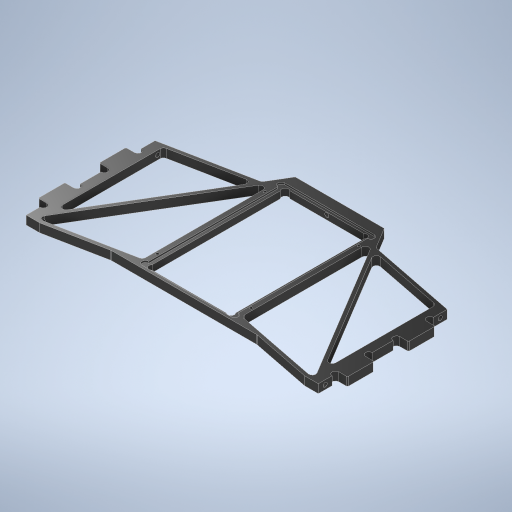
# Autodesk Inventor part: TorsoLowerFrame
Saved by Autodesk Inventor 2024.2 (Build 282272000, 272)
## iProperties
Created: 2024-01-11
Part Number: TorsoLowerFrame
Material: Aluminum 2014-T4
Document SubType Name: Modeling
Designer: Masato Kubotera
Density: 2.8 g/cm^3
Appearance: Glossy - Black
Vendor: meviy
Mass: 47.2837 g
Surface Area: 169.328 cm^2
Volume: 16.887 cm^3
Author: Masato Kubotera
Autodesk Inventor part; units mm, degrees
ref_plane "YZ Plane" through (0, 0, 0) normal (1, 0, 0) x (0, 1, 0)
ref_plane "XZ Plane" through (0, 0, 0) normal (0, 1, 0) x (-1, 0, 0)
sketch "Sketch1" plane through (0, 0, 0) normal (0, 0, 1) x (1, 0, 0)
  line L0 (-53, -85) -> (37.5, -85) construction
  line L1 (37.5, 85) -> (-53, 85) construction
  line L2 (0, -85) -> (0, 85) construction
  line L3 (-53, 0) -> (37.5, 0)
  line L4 (10, 90) -> (25.5, 90)
  line L5 (10, 90) -> (10, 85)
  arc A0 (6, 85) -> (10, 85) centre (8, 85) ccw
  line L6 (37.5, 85) -> (37.5, -85) construction
  line L7 (-53, -85) -> (-53, 85) construction
  line L8 (28.85, -25.8) -> (-53.75, -25.8) construction
  line L9 (-53.75, -25.8) -> (-53.75, 25.8) construction
  line L10 (-53.75, 25.8) -> (28.85, 25.8) construction
  line L11 (28.85, 25.8) -> (28.85, -25.8) construction
  line L12 (28.85, -25.8) -> (-53.75, 25.8) construction
  line L13 (-53.75, -25.8) -> (28.85, 25.8) construction
  line L14 (29.1, -26.05) -> (-54, -26.05)
  line L15 (-54, -26.05) -> (-54, 26.05)
  line L16 (-54, 26.05) -> (29.1, 26.05)
  line L17 (29.1, 26.05) -> (29.1, -26.05)
  line L18 (29.1, -26.05) -> (-54, 26.05) construction
  line L19 (-54, -26.05) -> (29.1, 26.05) construction
  line L20 (-52.5, 24.3) -> (27.6, 24.3) construction
  line L21 (27.6, 24.3) -> (27.6, -24.3) construction
  line L22 (27.6, -24.3) -> (-52.5, -24.3)
  line L23 (-52.5, -24.3) -> (-52.5, 24.3) construction
  line L24 (-52.5, 24.3) -> (27.6, -24.3) construction
  line L25 (27.6, 24.3) -> (-52.5, -24.3) construction
  line L26 (26.1724, 30.4098) -> (35.4616, 77.1098)
  line L27 (32.4688, 79.2137) -> (-45.1376, 32.5137)
  line L28 (-44.1064, 28.8) -> (24.2108, 28.8)
  line L29 (21.8631, 79.5) -> (-34.9135, 79.5)
  line L30 (37.5, 27.3) -> (-50.7865, 27.3) construction
  arc A1 (24.2108, 28.8) -> (26.1724, 30.4098) centre (24.2108, 30.8) ccw
  arc A2 (-45.1376, 32.5137) -> (-44.1064, 28.8) centre (-44.1064, 30.8) ccw
  arc A3 (22.8943, 75.7863) -> (21.8631, 79.5) centre (21.8631, 77.5) ccw
  arc A4 (29.1, 26.05) -> (25.1, 26.05) centre (27.1, 26.05) ccw
  arc A5 (27.6, 21.4716) -> (24.7716, 24.3) centre (26.1858, 22.8858) ccw
  arc A6 (-49.6716, 24.3) -> (-52.5, 21.4716) centre (-51.0858, 22.8858) ccw
  arc A7 (-50, 26.05) -> (-54, 26.05) centre (-52, 26.05) ccw
  circle A8 centre (18.85, 27.3) radius 1.5 construction
  circle A9 centre (18.85, 27.3) radius 1 construction
  line L31 (-12.45, -25.8) -> (-12.45, 25.7819) construction
  circle A10 centre (-43.75, 27.3) radius 1.5 construction
  circle A11 centre (-43.75, 27.3) radius 1 construction
  circle A12 centre (18.85, 27.3) radius 2.5 construction
  circle A13 centre (-43.75, 27.3) radius 2.5 construction
  line L32 (17.75, 90) -> (17.75, 85) construction
  line L33 (25.5, 90) -> (25.5, 85)
  arc A14 (25.5, 85) -> (29.5, 85) centre (27.5, 85) ccw
  line L34 (37.5, 85) -> (29.5, 85)
  line L35 (-10, 90) -> (-25.5, 90)
  line L36 (-10, 90) -> (-10, 85)
  arc A15 (-10, 85) -> (-6, 85) centre (-8, 85) ccw
  line L37 (-17.75, 90) -> (-17.75, 85) construction
  line L38 (-25.5, 90) -> (-25.5, 85)
  arc A16 (-29.5, 85) -> (-25.5, 85) centre (-27.5, 85) ccw
  line L39 (6, 85) -> (-6, 85)
  line L40 (33.5, 85) -> (33.5, 79) construction
  line L41 (-33.5, 85) -> (-33.5, 79) construction
  line L42 (-44.5951, 39.0791) -> (-36.875, 77.8902)
  line L43 (-41.6023, 36.9752) -> (22.8943, 75.7863)
  line L44 (-37.5, 85) -> (-29.5, 85)
  arc A17 (-44.5951, 39.0791) -> (-41.6023, 36.9752) centre (-42.6335, 38.6889) ccw
  arc A18 (-34.9135, 79.5) -> (-36.875, 77.8902) centre (-34.9135, 77.5) ccw
  line L45 (27.6, 0) -> (27.6, 21.4716)
  line L46 (24.7716, 24.3) -> (-49.6716, 24.3)
  line L47 (-52.5, 21.4716) -> (-52.5, 0)
  line L48 (-37.5, 85) -> (-47.6213, 34.1169)
  arc A19 (35.4616, 77.1098) -> (32.4688, 79.2137) centre (33.5, 77.5) ccw
  line L49 (-60, 25.9043) -> (-60, 0)
  line L50 (-60, 0) -> (-53, 0)
  line L51 (-60, 39.2) -> (-48.5, 39.2) construction
  line L52 (-48.5, 39.2) -> (-48.5, 44.2) construction
  line L53 (-48.5, 44.2) -> (-60, 44.2) construction
  line L54 (29.1, 26.05) -> (29.1, 20.1473)
  line L55 (-60, 25.9043) -> (-48.5516, 32.7934)
  line L56 (30.6, 0) -> (30.6, 42.2204)
  arc A20 (30.6384, 42.6106) -> (30.6, 42.2204) centre (32.6, 42.2204) ccw
  line L57 (37.5, 85) -> (37.5, 77.106)
  line L58 (37.5, 77.106) -> (30.6384, 42.6106)
  arc A21 (-48.5516, 32.7934) -> (-47.6213, 34.1169) centre (-49.5828, 34.5071) ccw
  point P0 (0, 0)
  point P1 (50, -85)
  point P2 (-47, 0)
  point P3 (-12.45, 0)
  point P4 (-49.0507, 0)
  point P5 (29.1, 0)
  point P6 (-20.5577, 28.8)
  point P7 (-52.5, 0)
  point P8 (27.6, 0)
  point P9 (24.6, 26.05)
  point P10 (-45.4774, 34.6434)
  point P11 (-36.5548, 79.5)
  point P12 (-52.5, 0)
  point P13 (27.6, 0)
  point P14 (0, 85)
  point P15 (-48.8888, 27.7448)
  point P16 (-60, 26.05)
  point P17 (-60, 24.5149)
  point P18 (-47.7938, 33.2495)
  point P19 (-54, 0)
  point P20 (-57, 0)
  dimension "d1" = 170
  dimension "d2" = 2
  dimension "d3" = 5
  dimension "d55" = 82.6
  dimension "d56" = 51.6
  dimension "d57" = 0.25
  dimension "d58" = 0.25
  dimension "d62" = 2
  dimension "d81" = 3
  dimension "d82" = 2
  dimension "d85" = 1.5
  dimension "d86" = 1.5
  dimension "d94" = 10
  dimension "d95" = 5
  dimension "d99" = 6
  dimension "d100" = 8
  dimension "d102" = 15.5
  dimension "d103" = 20
  dimension "d104" = 37.5
  dimension "d118" = 5.5
  dimension "d121" = 2
  dimension "d122" = 53
  dimension "d123" = 2
  dimension "d127" = 8.65
  dimension "d128" = 60
  dimension "d129" = 6
  dimension "d130" = 11.5
  dimension "d131" = 5
  dimension "d132" = 40.8
  dimension "d134" = 101.25
  dimension "d139" = 1.5
  dimension "d141" = 2
  dimension "d143" = 2
  constraints: 121 end point, 35 point on circle, 34 point on line, 22 centre point, 22 tangent, 20 symmetric about line, 15 midpoint, 11 equal radius, 10 horizontal, 10 parallel, 8 vertical, 5 coincident, 4 collinear, 3 perpendicular, 7 other
  measures "d1" distance of L1.start L0.end
  measures "d2" radius of A0
  measures "d3" distance of L4.start L5.end
  measures "d55" distance of L9.end L10.end
  measures "d56" distance of L8.end L9.end
  measures "d57" distance between parallel lines of L16 L10
  measures "d58" distance between parallel lines of L15 L9
  measures "d62" radius of A1
  measures "d81" diameter of A8
  measures "d82" diameter of A9
  measures "d85" distance between parallel lines of L10 L20
  measures "d86" distance between parallel lines of L21 L17
  measures "d94" horizontal distance of L10.end A8.centre
  measures "d95" diameter of A12
  measures "d99" distance of L40.start L40.end
  measures "d100" distance between parallel lines of L33 L40
  measures "d102" distance of L4.start L4.end
  measures "d103" distance between parallel lines of L36 L5
  measures "d104" distance between parallel lines of L6 L2
  measures "d118" distance between parallel lines of L1 L29
  measures "d121" distance between parallel lines of L42 L48
  measures "d122" distance of point (0, 85) L1.end
  measures "d123" distance between parallel lines of L27 L43
  measures "d127" distance between parallel lines of L6 L11
  measures "d128" distance between parallel lines of L49 L2
  measures "d129" distance between parallel lines of L15 L49
  measures "d130" distance of L51.start L51.end
  measures "d131" distance of L51.end L52.end
  measures "d132" distance between parallel lines of L53 L1
  measures "d134" angle of L42 L29
  measures "d139" distance between parallel lines of L56 L17
  measures "d141" distance between parallel lines of L58 L26
  measures "d143" distance edge to line of A19 L6
extrude "Extrusion1" add sketch "Sketch1" against normal blind 5 contours L50 L15 L16 L17 L3 L45 A5 L46 A6 L47 | L50 L49 L55 A21 L48 L44 A16 L38 L35 L36 A15 L39 A0 L5 L4 L33 A14 L34 L57 L58 A20 L56 L3 L17 A4 L16 A7 L15 | A7 L16 | A4 L16
extrude "Extrusion2" cut sketch "Sketch1" against normal blind 1 contours L50 L15 L16 L17 L3 L45 A5 L46 A6 L47 | L3 L17 L14 L15 L50 | L47 A6 L46 A5 L45 L3 | A7 L16 | A4 L16
hole "M2" at (18.85, 27.3, 0) at (-43.75, 27.3, 0) direction (0, 0, -1) diameter 1.567 end through all thread size "M2x0.4" class "6H" standard "ANSI Metric M Profile"
sketch "Sketch6" plane through (29.5, 85, 0) normal (0, 1, 0) x (1, 0, 0)
  line L0 (0, 5) -> (8, 5) projected
  line L1 (4, 5) -> (4, 0)
  line L2 (8, 0) -> (0, 0) projected
  line L3 (-63, 5) -> (-63, 0)
  line L4 (-67, 5) -> (-59, 5) projected
  point P0 (-29.5, 0)
  point P1 (-86, 5)
  point P2 (-86, 0)
  point P3 (4, 0)
  point P4 (-63, 0)
  point P5 (4, 2.5)
  point P6 (-63, 2.5)
  constraints: 4 end point, 4 midpoint, 2 vertical
hole "SideーM3" at (33.5, 85, -2.5) at (-33.5, 85, -2.5) direction (0, -1, 0) diameter 2.459 depth 10 thread size "M3x0.5" class "6H" standard "ANSI Metric M Profile"
chamfer "C0.5" distance 0.5 angle 45 4 edges at (25.5, 90, -2.5) (10, 90, -2.5) (-10, 90, -2.5) (-25.5, 90, -2.5)
mirror "Mirror5" about plane through (0, 0, 0) normal (0, 1, 0)
ref_plane "Work Plane1" through (-12.45, 21.4716, -1) normal (1, 0, 0) x (0, 0, -1)
sketch "Sketch7" plane through (-60, 25.9043, -5) normal (-1, 0, 0) x (0, 0, 1)
  line L0 (5, -25.9043) -> (0, -25.9043)
  line L1 (0, 0) -> (0, -51.8087) projected
  point P0 (2.5, -25.9043)
  point P1 (2.5, -25.9043)
  constraints: 2 end point, 2 midpoint, 1 coincident
hole "Back-M3" at (-60, 0, -2.5) direction (1, 0, 0) diameter 2.459 depth 7.5 thread size "M3x0.5" class "6H" standard "ANSI Metric M Profile"
body "Solid1"
